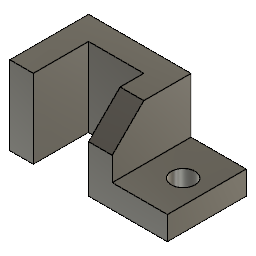
ch2Example-Video v2 (Autodesk Fusion 360 design; units mm, degrees)
Autodesk Fusion 360 part; units mm, degrees
sketch "Sketch1" plane through (0, 0, 0) normal (0, 1, 0) x (1, 0, 0) in component "Component"
  line L0 (0, -63.5) -> (0, 0)
  line L1 (0, 0) -> (63.5, 0)
  line L2 (63.5, 0) -> (63.5, -19.05)
  line L3 (63.5, -19.05) -> (19.05, -19.05)
  line L4 (19.05, -19.05) -> (19.05, -63.5)
  line L5 (19.05, -63.5) -> (0, -63.5)
  dimension "d1" = 63.5
  dimension "d2" = 19.05
  dimension "d3" = 19.05
  dimension "d4" = 63.5
  constraint vertical L0
  constraint perpendicular L0 L1
  constraint perpendicular L1 L2
  constraint perpendicular L2 L3
  constraint perpendicular L3 L4
  constraint perpendicular L0 L5
  constraint coincident L0.end L1.start
  measures "d1" distance of L0.end L1.end
  measures "d2" distance of L1.end L2.end
  measures "d3" distance of L0.start L4.end
  measures "d4" distance of L0.start L0.end
extrude "Extrude1" add sketch "Sketch1" along normal blind 63.5 in component "Component"
sketch "Sketch2" plane through (0, 0, 63.5) normal (0, 0, 1) x (-1, 0, 0) in component "Component"
  line L0 (0, 0) -> (-19.05, 0)
  line L1 (-19.05, 0) -> (-19.05, -63.5)
  line L2 (-19.05, -63.5) -> (0, -63.5)
  line L3 (0, -63.5) -> (0, 0)
  line L4 (0, -63.5) -> (63.5, -63.5)
  line L5 (63.5, -63.5) -> (63.5, 0)
  line L6 (63.5, 0) -> (44.45, 0)
  line L7 (44.45, 0) -> (44.45, -44.45)
  line L8 (44.45, -44.45) -> (0, -44.45)
  line L9 (0, -63.5) -> (0, -44.45)
  dimension "d7" = 19.05
  dimension "d8" = 63.5
  dimension "d9" = 63.5
  dimension "d10" = 19.05
  constraint coincident L2.end L3.start
  constraint perpendicular L3 L4
  constraint perpendicular L2 L5
  constraint perpendicular L5 L6
  constraint perpendicular L6 L7
  constraint coincident L3 L8.end
  constraint perpendicular L3 L8
  measures "d7" distance of L4 L8
  measures "d8" distance of L2.end L4.end
  measures "d9" distance of L4.end L5.end
  measures "d10" distance of L5.end L6.end
extrude "Extrude2" add sketch "Sketch2" against normal blind 63.5 contours L3 L4 L5 L6 L7 L8 L9 in component "Component"
sketch "Sketch3" plane through (0, 0, 19.05) normal (0, 0, 1) x (-1, 0, 0) in component "Component"
  line L0 (-19.05, 0) -> (-63.5, 0)
  line L1 (-63.5, 0) -> (-63.5, -63.5)
  line L2 (-63.5, -63.5) -> (-19.05, -63.5)
  line L3 (-19.05, -63.5) -> (-19.05, 0)
  circle A0 centre (-44.45, -31.75) radius 9.525
  dimension "d13" = 19.05
  dimension "d14" = 31.75
  dimension "d15" = 19.05
  measures "d13" diameter of A0
  measures "d14" distance of L2 A0.centre
  measures "d15" distance of L1 A0.centre
extrude "Extrude3" cut sketch "Sketch3" against normal through all contours A0 in component "Component"
sketch "Sketch4" plane through (19.05, 0, 0) normal (1, 0, 0) x (0, 1, 0) in component "Component"
  line L0 (0, 63.5) -> (0, 19.05)
  line L1 (0, 19.05) -> (63.5, 19.05)
  line L2 (63.5, 19.05) -> (63.5, 63.5)
  line L3 (63.5, 63.5) -> (0, 63.5)
  line L4 (25.4, 63.5) -> (0, 38.1)
  dimension "d17" = 45
  dimension "d18" = 25.4
  constraint coincident L3 L4.start
  constraint coincident L0 L4.end
  measures "d17" angle of L3 L4
  measures "d18" distance of L0.start L4.start
extrude "Extrude4" cut sketch "Sketch4" against normal up to surface (19.05 mm away) contours L0 L3 L4 in component "Component"
component "Component" placed x (1, 0, 0) y (0, 1, 0) z (0, 0, 1) at (0, 0, 0)
